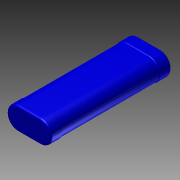
# Autodesk Inventor part: 276-1491
Saved by Autodesk Inventor 2013 (Build 170138000, 138)
## iProperties
Category: Power
Company: Autodesk Inc.
Created: 2012-02-01
Part Number: 276-1491
Document SubType Name: Modeling
Designer: Autodesk Inc.
Density: 1 g/cm^3
Catalog Web Link: http://www.vexrobotics.com/products/accessories/power/276-1491.html
Vendor: VEX
Material: Generic
Author: Autodesk Inc.
Autodesk Inventor part; units mm, degrees
ref_plane "YZ Plane" through (0, 0, 0) normal (1, 0, 0) x (0, 1, 0)
ref_plane "XZ Plane" through (0, 0, 0) normal (0, 1, 0) x (-1, 0, 0)
ref_plane "XY Plane" through (0, 0, 0) normal (0, 0, 1) x (1, 0, 0)
sketch "Sketch1" plane through (0, 0, 0) normal (0, 0, 1) x (1, 0, 0)
  arc A0 (-11.811, 11.811) -> (-11.811, -11.811) centre (-11.811, 0) ccw
  line L0 (-11.811, 11.811) -> (11.811, 11.811)
  arc A1 (11.811, -11.811) -> (11.811, 11.811) centre (11.811, 0) ccw
  line L1 (11.811, -11.811) -> (-11.811, -11.811)
  point P0 (0, 0)
  point P1 (0, 0)
  constraints: 4 end point, 4 point on circle, 2 centre point
extrude "Extrusion1" add sketch "Sketch1" along normal mid plane 105.41
sketch "Sketch2" plane through (0, 0, 52.705) normal (0, 0, 1) x (1, 0, 0)
  arc A0 (11.811, -12.319) -> (11.811, 12.319) centre (11.811, 0) ccw
  line L0 (11.811, -12.319) -> (-11.811, -12.319)
  arc A1 (-11.811, 12.319) -> (-11.811, -12.319) centre (-11.811, 0) ccw
  line L1 (-11.811, 12.319) -> (11.811, 12.319)
  point P0 (0, 0)
  point P1 (0, 0)
  constraints: 4 end point, 4 point on circle, 2 centre point
extrude "Extrusion2" add sketch "Sketch2" along normal blind 12.954
fillet "Fillet1" radius 2.032 4 edges at (-24.13, 0, 65.659) (0, 12.319, 65.659) (24.13, 0, 65.659) (0, -12.319, 65.659)
chamfer "Chamfer1" distance 0.508 angle 45 4 edges at (0, 12.319, 52.705) (24.13, 0, 52.705) (0, -12.319, 52.705) (-24.13, 0, 52.705)
mirror "Mirror1" about plane through (0, 0, 0) normal (0, 0, 1) of "Extrusion2", "Fillet1", "Chamfer1"
sketch "Sketch3" plane through (0, 0, 65.659) normal (0, 0, 1) x (1, 0, 0)
  line L0 (11.811, 5.969) -> (-11.811, 5.969)
  arc A0 (11.811, -5.969) -> (11.811, 5.969) centre (11.811, 0) ccw
  line L1 (-11.811, -5.969) -> (11.811, -5.969)
  arc A1 (-11.811, 5.969) -> (-11.811, -5.969) centre (-11.811, 0) ccw
  point P0 (0, 0)
  point P1 (11.811, 0)
  point P2 (-11.811, 0)
  point P3 (0, 0)
  constraints: 4 end point, 4 point on circle, 2 centre point
extrude "Extrusion3" add sketch "Sketch3" along normal blind 1.905 draft -30
fillet "Fillet2" radius 0.635 4 edges at (0, 4.8691, 67.564) (16.6801, 0, 67.564) (0, -4.8691, 67.564) (-16.6801, 0, 67.564)
body "Solid1"
